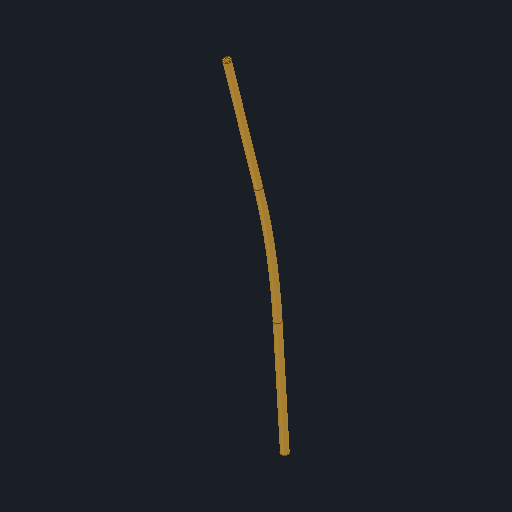
# Autodesk Inventor part: prop_shaft
Saved by Autodesk Inventor 2023 (Build 270158030, 158C)
## iProperties
Created: 2022-04-18
Part Number: prop_shaft
Material: Generic
Document SubType Name: Modeling
Designer: kardo
Density: 1 g/cm^3
Appearance: Brass - Prop shaft
Author: kardo
Autodesk Inventor part; units mm, degrees
ref_plane "YZ Plane" through (0, 0, 0) normal (1, 0, 0) x (0, 1, 0)
ref_plane "XZ Plane" through (0, 0, 0) normal (0, 1, 0) x (-1, 0, 0)
ref_plane "XY Plane" through (0, 0, 0) normal (0, 0, 1) x (1, 0, 0)
derived "stencil_frame.ipt"
sketch "sk_drivetrain_profile" plane through (6, 0, 0) normal (1, 0, 0) x (0, 1, 0)
  line L0 (-547.3485, 0) -> (393.091, 0) construction
  line L1 (-363, 4592.9714) -> (-363, -1605.7041) construction
  line L2 (0, 4592.9714) -> (0, -1605.7041) construction
  line L3 (-140.2591, 52.979) -> (-133.4853, 25.8107)
  line L4 (-388, 0) -> (-343.0839, 2.7472)
  line L5 (-136.8722, 39.3948) -> (-222.489, 18.0482)
  line L6 (-307.9329, 4.8971) -> (-264.6067, 7.5471) construction
  line L7 (-264.6067, 7.5471) -> (-222.489, 18.0482) construction
  line L8 (-133.4853, 25.8107) -> (-133.4853, 20.8107) construction
  line L9 (-343.0839, 2.7472) -> (-307.9329, 4.8971)
  line L10 (-1229.7832, 4422.8213) -> (280.3081, -1633.8241) construction
  line L11 (-223.0651, 20.3587) -> (-137.4483, 41.7054) construction
  line L12 (-136.2962, 37.0843) -> (-221.913, 15.7377) construction
  line L13 (-223.0651, 20.3587) -> (-221.913, 15.7377) construction
  spline S0 degree 2 poles (-307.9329, 4.8971) (-264.6067, 7.5471) (-222.489, 18.0482) knots 1 1 1 2 2 2
  line L14 (0, 18.496) -> (-254.1001, 20.6178) construction
  line L15 (-55.3282, 20.1581) -> (-309.4681, 22.2802) construction
  point P0 (0, 0)
  point P1 (-213.541, 20.2792)
  point P2 (-204.017, 20.1996)
  point P3 (-199.3598, 21.3608)
ref_plane "plane_motor_mount" through (0, -127.05, 0) normal (0, 0.9702957, 0.2419219) x (-1, 0, 0)
sketch "sk_prop_shaft_profile" plane through (0, -127.05, 0) normal (0, 0.9702957, 0.2419219) x (-1, 0, 0)
  circle A0 centre (-6, 40.6009) radius 2.3812
  point P0 (0, -30.7362)
  dimension "d1" = 4.7625
  constraints: 1 centre point, 1 coincident
  measures "d1" diameter of A0
derived "parameters_powertrain.ipt"
sweep "Sweep1" add profiles "sk_prop_shaft_profile" path "sk_drivetrain_profile" path curves L5 S0 L9 L4
shell "Shell1" thickness 0.7937 removed faces 2 at (6.4028, -388.0321, 0.5254) at (6.0476, -136.967, 39.7748)
equation "\"d1\" = prop_shaft_od"
equation "\"prop_shaft_od\" = 4.7625"
body "Solid1"
